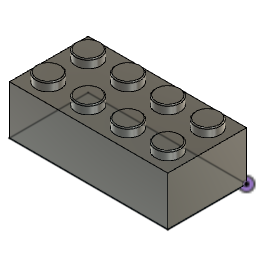
ToyBlockv2 (Autodesk Fusion 360 design; units mm, degrees)
part number: 2025-05-08-20-50-47-826
part number: 2025-05-08-20-52-24-790
Autodesk Fusion 360 part; units mm, degrees
note: some values were not read from the file. Set by a fixed rule: which sketch regions a step uses.
sketch "Sketch1" plane through (0, 0, 0) normal (0, 0, 1) x (1, 0, 0) in component "2x8 Block"
  line L0 (0, 0) -> (-31.8, 0)
  line L1 (-31.8, 0) -> (-31.8, -15.8)
  line L2 (-31.8, -15.8) -> (0, -15.8)
  line L3 (0, -15.8) -> (0, 0)
  dimension "d1" = 31.8
  dimension "d2" = 15.8
  constraint horizontal L0
  constraint vertical L1
  constraint horizontal L2
  constraint vertical L3
  constraint coincident L0.start L3.end
  measures "d1" distance of L0.start L0.end
  measures "d2" distance of L0.start L2.end
extrude "Extrude2" add sketch "Sketch1" along normal blind 9.8 makes body 1 in component "2x8 Block"
sketch "Sketch2" plane through (0, 0, 9.8) normal (0, 0, 1) x (-1, 0, 0) in component "2x8 Block"
  line L0 (0, 15.8) -> (0, 0)
  line L1 (0, 0) -> (31.8, 0)
  line L2 (31.8, 0) -> (31.8, 15.8)
  line L3 (31.8, 15.8) -> (0, 15.8)
  circle A0 centre (3.9, 11.9) radius 2.5
  dimension "d7" = 5
  dimension "d8" = 3.9
  dimension "d9" = 3.9
  measures "d7" diameter of A0
  measures "d8" vertical distance of L0.start A0.centre
  measures "d9" horizontal distance of L0.start A0.centre
extrude "Extrude3" add sketch "Sketch2" along normal blind 1.7 contours A0 bodies 1 in component "2x8 Block"
pattern_linear "R-Pattern1" count 2 spacing 8 along (0, 1, 0) count 4 spacing 8 along (-1, 0, 0) of "Extrude3" in component "2x8 Block"
shell "Shell1" thickness 1.49 removed faces 1 at (-21.2, -10.5333, 0) on bodies 1 in component "2x8 Block"
sketch "Sketch3" plane through (0, 0, 0) normal (0, 0, 1) x (1, 0, 0) in component "2x8 Block"
  line L0 (-19.8337, -11.8825) -> (-27.8704, -3.7331)
  circle A0 centre (-23.8521, -7.8078) radius 3.15
  circle A1 centre (-23.8521, -7.8078) radius 2.15
  circle A2 centre (-23.8521, -7.8078) radius 4.15
  dimension "d17" = 6.3
  dimension "d18" = -1
  dimension "d19" = 1
  constraint midpoint L0 A0.centre
  measures "d17" diameter of A0
extrude "Extrude4" add sketch "Sketch3" along normal blind 8.1 separate body contours L0 A0 A1 | L0 A0 A1 makes body 2 in component "2x8 Block"
pattern_linear "R-Pattern2" count 3 spacing 8 along (1, 0, 0) of "Extrude4" makes body 3 makes body 4 in component "2x8 Block"
fillet "Fillet5" radius 0.2 8 edges at (-25.5692, -2.996, 11.5) (-25.5692, -10.996, 11.5) (-17.5692, -10.996, 11.5) (-17.5692, -2.996, 11.5) (-9.5692, -2.996, 11.5) (-9.5692, -10.996, 11.5) (-1.5692, -2.996, 11.5) (-1.5692, -10.996, 11.5) on bodies 1 in component "2x8 Block"
component "2x8 Block" placed x (1, 0, 0) y (0, 1, 0) z (0, 0, 1) at (0, 0, 0)
named bodies: "Body"
